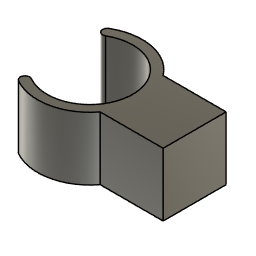
Wardrobe Leg Holders V2 (Autodesk Fusion 360 design; units mm, degrees)
Autodesk Fusion 360 part; units mm, degrees
sketch "Sketch1" plane through (0, 0, 0) normal (0, 0, 1) x (1, 0, 0)
  arc A0 (-6.8, -11.7779) -> (-6.8, 11.7779) centre (0, 0) ccw
  line L0 (0, 0) -> (-6.8, -11.7779) construction
  line L1 (0, 0) -> (-6.8, 11.7779) construction
  arc A1 (-8.3, -14.376) -> (-8.3, 14.376) centre (0, 0) ccw
  arc A2 (-8.3, 14.376) -> (-6.8, 11.7779) centre (-7.55, 13.077) ccw
  arc A3 (-6.8, -11.7779) -> (-8.3, -14.376) centre (-7.55, -13.077) ccw
  line L2 (13.2499, 10) -> (33.2499, 10)
  line L3 (33.2499, 10) -> (33.2499, -10)
  line L4 (33.2499, -10) -> (13.2499, -10)
  line L5 (13.2499, -10) -> (13.2499, -3.0659)
  line L6 (13.2499, 3.0659) -> (13.2499, 10)
  dimension "d1" = 13.6
  dimension "d2" = 120
  dimension "d3" = 3
  dimension "d4" = 20
  dimension "d5" = 20
  constraint coincident A0.centre L0.start
  constraint vertical A0.start A0.end
  constraint tangent A1 A2
  constraint tangent A1 A3
  constraint vertical A2.centre A3.centre
  constraint tangent A0 A2
  constraint horizontal L2
  constraint vertical L3
  constraint horizontal L4
  constraint vertical L5
  constraint coincident A1 L4.end
  constraint coincident A1 L2.start
  constraint coincident A0 L5.end
  constraint coincident A0 L6.start
  constraint collinear L5 L6
  measures "d1" radius of A0
  measures "d2" angle of L0 L1
  measures "d4" distance of L2.start L2.end
  measures "d5" distance of L2.start L4.end
extrude "Extrude1" add sketch "Sketch1" along normal blind 20
